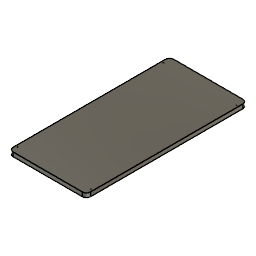
Tapa encapsulado (Autodesk Fusion 360 design; units mm, degrees)
part number: 2026-06-22-14-09-30-077
Autodesk Fusion 360 part; units mm, degrees
sketch "Boceto1" plane through (0, 0, 0) normal (0, 0, 1) x (1, 0, 0)
  line L0 (46.5, -96.4) -> (-46.5, -96.4)
  line L1 (-46.5, -96.4) -> (-46.5, 96.4)
  line L2 (-46.5, 96.4) -> (46.5, 96.4)
  line L3 (46.5, 96.4) -> (46.5, -96.4)
  line L4 (46.5, -96.4) -> (-46.5, 96.4) construction
  line L5 (-46.5, -96.4) -> (46.5, 96.4) construction
  dimension "d1" = 93
  dimension "d2" = 192.8
  constraint horizontal L0
  constraint perpendicular L0 L1
  constraint parallel L0 L2
  constraint parallel L1 L3
  constraint coincident L4 origin
  constraint coincident L5 origin
  measures "d1" distance of L1.end L2.end
  measures "d2" distance of L0.end L1.end
extrude "Extruir1" add sketch "Boceto1" along normal blind 5
fillet "Empalme1" radius 5 1 edges at (-46.5, 96.4, 2.5)
fillet "Empalme2" radius 5 1 edges at (46.5, 96.4, 2.5)
fillet "Empalme3" radius 5 1 edges at (46.5, -96.4, 2.5)
fillet "Empalme4" radius 5 1 edges at (-46.5, -96.4, 2.5)
sketch "Boceto2" plane through (0, 0, 5) normal (0, 0, 1) x (-1, 0, 0)
  arc A0 (46.5, 91.4) -> (41.5, 96.4) centre (41.5, 91.4) ccw
  line L0 (41.5, 96.4) -> (-41.5, 96.4)
  arc A1 (-41.5, 96.4) -> (-46.5, 91.4) centre (-41.5, 91.4) ccw
  line L1 (-46.5, 91.4) -> (-46.5, -91.4)
  arc A2 (-46.5, -91.4) -> (-41.5, -96.4) centre (-41.5, -91.4) ccw
  line L2 (-41.5, -96.4) -> (41.5, -96.4)
  arc A3 (41.5, -96.4) -> (46.5, -91.4) centre (41.5, -91.4) ccw
  line L3 (46.5, -91.4) -> (46.5, 91.4)
  line L4 (-46.5, -96.4) -> (-46.5, -86.4)
  line L5 (-46.5, -86.4) -> (-44, -86.4)
  line L6 (-44, -86.4) -> (44, -86.4)
  line L7 (44, -86.4) -> (44, 88.6)
  line L8 (44, 88.6) -> (-44, 88.6)
  line L9 (-44, 88.6) -> (-44, -86.4)
  dimension "d13" = 10
  dimension "d14" = 2.5
  dimension "d15" = 88
  dimension "d16" = 175
  dimension "d17" = 88
  constraint parallel L1 L4
  constraint perpendicular L1 L5
  constraint perpendicular L1 L6
  constraint perpendicular L6 L7
  constraint perpendicular L1 L8
  measures "d13" distance of L4.start L4.end
  measures "d14" distance of L4.end L5.end
  measures "d15" distance of L5.end L6.end
  measures "d16" distance of L6.end L7.end
  measures "d17" distance of L7.end L8.end
hole "Agujero1" at (-44, -88.6, 5) at (-44, 86.4, 5) at (44, 86.4, 5) at (44, -88.6, 5) direction (0, 0, -1) diameter 0.769 depth 5 tip angle 118
thread "Rosca1" "ISO Metric profile 1.0 M1x0.25 M1x0.25 6H" thread offset 0 thread depth 7.4
